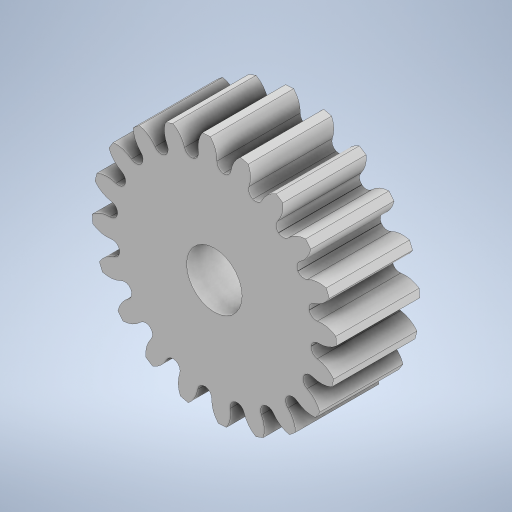
# Autodesk Inventor part: Spur_Gear_20
Saved by Autodesk Inventor 2024 (Build 280153000, 153)
## iProperties
Created: 2024-10-23
Part Number: Spur_Gear_20
Material: Generic
Document SubType Name: Modeling
Designer: Yash Purswani
Density: 1 g/cm^3
Appearance: Default
Author: Yash Purswani
Autodesk Inventor part; units mm, degrees
ref_plane "YZ Plane" through (0, 0, 0) normal (1, 0, 0) x (0, 1, 0)
ref_plane "XZ Plane" through (0, 0, 0) normal (0, 1, 0) x (-1, 0, 0)
ref_plane "XY Plane" through (0, 0, 0) normal (0, 0, 1) x (1, 0, 0)
sketch "Sketch1" plane through (0, 0, 0) normal (0, 0, 1) x (1, 0, 0)
  line L0 (-0.0011, 22.0023) -> (-0.0011, 20.9337)
  arc A0 (0.4688, 18.788) -> (-0.7145, 21.9884) centre (-4.1398, 18.903) ccw
  arc A1 (-2.1725, 21.8925) -> (-2.8834, 18.5713) centre (1.6629, 19.3348) ccw
  arc A2 (-3.8684, 17.0671) -> (-2.8834, 18.5713) centre (-4.1544, 18.3289) ccw
  arc A3 (0.4688, 18.788) -> (1.6392, 17.4231) centre (1.7604, 18.7112) ccw
  arc A4 (-8.8313, 20.1496) -> (-8.4812, 16.7714) centre (-4.3933, 18.9023) ccw
  arc A5 (-5.36, 18.0133) -> (-7.4743, 20.6914) centre (-9.7785, 16.6986) ccw
  arc A6 (-5.36, 18.0133) -> (-3.8251, 17.0768) centre (-4.1079, 18.3394) ccw
  arc A7 (-8.9531, 15.0364) -> (-8.4812, 16.7714) centre (-9.615, 16.1481) ccw
  arc A8 (-14.6257, 16.4344) -> (-13.2487, 13.3297) centre (-10.0194, 16.6196) ccw
  arc A9 (-10.6641, 15.4754) -> (-13.5025, 17.369) centre (-14.4601, 12.8596) ccw
  arc A10 (-10.6641, 15.4754) -> (-8.9149, 15.059) centre (-9.574, 16.1724) ccw
  arc A11 (-13.1614, 11.5338) -> (-13.2487, 13.3297) centre (-14.1344, 12.3865) ccw
  arc A12 (-18.9883, 11.1105) -> (-16.7194, 8.5832) centre (-14.6647, 12.71) ccw
  arc A13 (-14.9243, 11.4226) -> (-18.209, 12.3464) centre (-17.7262, 7.7618) ccw
  arc A14 (-14.9243, 11.4226) -> (-13.1321, 11.5671) centre (-14.103, 12.4223) ccw
  arc A15 (-16.0813, 6.9022) -> (-16.7194, 8.5832) centre (-17.2703, 7.4125) ccw
  arc A16 (-21.4923, 4.699) -> (-18.5534, 2.9965) centre (-17.8746, 7.5563) ccw
  arc A17 (-17.7236, 6.2517) -> (-21.133, 6.1153) centre (-19.2571, 1.9042) ccw
  arc A18 (-17.7236, 6.2517) -> (-16.0638, 6.943) centre (-17.2515, 7.4563) ccw
  arc A19 (-17.4272, 1.595) -> (-18.5534, 2.9965) centre (-18.7156, 1.7129) ccw
  arc A20 (-21.8925, -2.1725) -> (-18.5713, -2.8834) centre (-19.3348, 1.6629) ccw
  arc A21 (-18.788, 0.4688) -> (-21.9884, -0.7145) centre (-18.903, -4.1398) ccw
  arc A22 (-18.788, 0.4688) -> (-17.4231, 1.6392) centre (-18.7112, 1.7604) ccw
  arc A23 (-17.0671, -3.8684) -> (-18.5713, -2.8834) centre (-18.3289, -4.1544) ccw
  arc A24 (-20.1496, -8.8313) -> (-16.7714, -8.4812) centre (-18.9023, -4.3933) ccw
  arc A25 (-18.0133, -5.36) -> (-20.6914, -7.4743) centre (-16.6986, -9.7785) ccw
  arc A26 (-18.0133, -5.36) -> (-17.0768, -3.8251) centre (-18.3394, -4.1079) ccw
  arc A27 (-15.0364, -8.9531) -> (-16.7714, -8.4812) centre (-16.1481, -9.615) ccw
  arc A28 (-16.4344, -14.6257) -> (-13.3297, -13.2487) centre (-16.6196, -10.0194) ccw
  arc A29 (-15.4754, -10.6641) -> (-17.369, -13.5025) centre (-12.8596, -14.4601) ccw
  arc A30 (-15.4754, -10.6641) -> (-15.059, -8.9149) centre (-16.1724, -9.574) ccw
  arc A31 (-11.5338, -13.1614) -> (-13.3297, -13.2487) centre (-12.3865, -14.1344) ccw
  arc A32 (-11.1105, -18.9883) -> (-8.5832, -16.7194) centre (-12.71, -14.6647) ccw
  arc A33 (-11.4226, -14.9243) -> (-12.3464, -18.209) centre (-7.7618, -17.7262) ccw
  arc A34 (-11.4226, -14.9243) -> (-11.5671, -13.1321) centre (-12.4223, -14.103) ccw
  arc A35 (-6.9022, -16.0813) -> (-8.5832, -16.7194) centre (-7.4125, -17.2703) ccw
  arc A36 (-4.699, -21.4923) -> (-2.9965, -18.5534) centre (-7.5563, -17.8746) ccw
  arc A37 (-6.2517, -17.7236) -> (-6.1153, -21.133) centre (-1.9042, -19.2571) ccw
  arc A38 (-6.2517, -17.7236) -> (-6.943, -16.0638) centre (-7.4563, -17.2515) ccw
  arc A39 (-1.595, -17.4272) -> (-2.9965, -18.5534) centre (-1.7129, -18.7156) ccw
  arc A40 (2.1725, -21.8925) -> (2.8834, -18.5713) centre (-1.6629, -19.3348) ccw
  arc A41 (-0.4688, -18.788) -> (0.7145, -21.9884) centre (4.1398, -18.903) ccw
  arc A42 (-0.4688, -18.788) -> (-1.6392, -17.4231) centre (-1.7604, -18.7112) ccw
  arc A43 (3.8684, -17.0671) -> (2.8834, -18.5713) centre (4.1544, -18.3289) ccw
  arc A44 (8.8313, -20.1496) -> (8.4812, -16.7714) centre (4.3933, -18.9023) ccw
  arc A45 (5.36, -18.0133) -> (7.4743, -20.6914) centre (9.7785, -16.6986) ccw
  arc A46 (5.36, -18.0133) -> (3.8251, -17.0768) centre (4.1079, -18.3394) ccw
  arc A47 (8.9531, -15.0364) -> (8.4812, -16.7714) centre (9.615, -16.1481) ccw
  arc A48 (14.6257, -16.4344) -> (13.2487, -13.3297) centre (10.0194, -16.6196) ccw
  arc A49 (10.6641, -15.4754) -> (13.5025, -17.369) centre (14.4601, -12.8596) ccw
  arc A50 (10.6641, -15.4754) -> (8.9149, -15.059) centre (9.574, -16.1724) ccw
  arc A51 (13.1614, -11.5338) -> (13.2487, -13.3297) centre (14.1344, -12.3865) ccw
  arc A52 (18.9883, -11.1105) -> (16.7194, -8.5832) centre (14.6647, -12.71) ccw
  arc A53 (14.9243, -11.4226) -> (18.209, -12.3464) centre (17.7262, -7.7618) ccw
  arc A54 (14.9243, -11.4226) -> (13.1321, -11.5671) centre (14.103, -12.4223) ccw
  arc A55 (16.0813, -6.9022) -> (16.7194, -8.5832) centre (17.2703, -7.4125) ccw
  arc A56 (21.4923, -4.699) -> (18.5534, -2.9965) centre (17.8746, -7.5563) ccw
  arc A57 (17.7236, -6.2517) -> (21.133, -6.1153) centre (19.2571, -1.9042) ccw
  arc A58 (17.7236, -6.2517) -> (16.0638, -6.943) centre (17.2515, -7.4563) ccw
  arc A59 (17.4272, -1.595) -> (18.5534, -2.9965) centre (18.7156, -1.7129) ccw
  arc A60 (21.8925, 2.1725) -> (18.5713, 2.8834) centre (19.3348, -1.6629) ccw
  arc A61 (18.788, -0.4688) -> (21.9884, 0.7145) centre (18.903, 4.1398) ccw
  arc A62 (18.788, -0.4688) -> (17.4231, -1.6392) centre (18.7112, -1.7604) ccw
  arc A63 (17.0671, 3.8684) -> (18.5713, 2.8834) centre (18.3289, 4.1544) ccw
  arc A64 (20.1496, 8.8313) -> (16.7714, 8.4812) centre (18.9023, 4.3933) ccw
  arc A65 (18.0133, 5.36) -> (20.6914, 7.4743) centre (16.6986, 9.7785) ccw
  arc A66 (18.0133, 5.36) -> (17.0768, 3.8251) centre (18.3394, 4.1079) ccw
  arc A67 (15.0364, 8.9531) -> (16.7714, 8.4812) centre (16.1481, 9.615) ccw
  arc A68 (16.4344, 14.6257) -> (13.3297, 13.2487) centre (16.6196, 10.0194) ccw
  arc A69 (15.4754, 10.6641) -> (17.369, 13.5025) centre (12.8596, 14.4601) ccw
  arc A70 (15.4754, 10.6641) -> (15.059, 8.9149) centre (16.1724, 9.574) ccw
  arc A71 (11.5338, 13.1614) -> (13.3297, 13.2487) centre (12.3865, 14.1344) ccw
  arc A72 (11.1105, 18.9883) -> (8.5832, 16.7194) centre (12.71, 14.6647) ccw
  arc A73 (11.4226, 14.9243) -> (12.3464, 18.209) centre (7.7618, 17.7262) ccw
  arc A74 (11.4226, 14.9243) -> (11.5671, 13.1321) centre (12.4223, 14.103) ccw
  arc A75 (6.9022, 16.0813) -> (8.5832, 16.7194) centre (7.4125, 17.2703) ccw
  arc A76 (4.699, 21.4923) -> (2.9965, 18.5534) centre (7.5563, 17.8746) ccw
  arc A77 (6.2517, 17.7236) -> (6.1153, 21.133) centre (1.9042, 19.2571) ccw
  arc A78 (6.2517, 17.7236) -> (6.943, 16.0638) centre (7.4563, 17.2515) ccw
  arc A79 (1.595, 17.4272) -> (2.9965, 18.5534) centre (1.7129, 18.7156) ccw
  arc A80 (20.6914, 7.4743) -> (20.1496, 8.8313) centre (0, 0) ccw
  arc A81 (-17.0768, -3.8251) -> (-17.0671, -3.8684) centre (0, 0) ccw
  arc A82 (-17.4231, 1.6392) -> (-17.4272, 1.595) centre (0, 0) ccw
  arc A83 (-16.0638, 6.943) -> (-16.0813, 6.9022) centre (0, 0) ccw
  arc A84 (-13.1321, 11.5671) -> (-13.1614, 11.5338) centre (0, 0) ccw
  arc A85 (17.4231, -1.6392) -> (17.4272, -1.595) centre (0, 0) ccw
  arc A86 (17.0768, 3.8251) -> (17.0671, 3.8684) centre (0, 0) ccw
  arc A87 (15.059, 8.9149) -> (15.0364, 8.9531) centre (0, 0) ccw
  arc A88 (11.5671, 13.1321) -> (11.5338, 13.1614) centre (0, 0) ccw
  arc A89 (-0.0011, 22) -> (-2.1725, 21.8925) centre (0, 0) ccw
  arc A90 (6.1153, 21.133) -> (4.699, 21.4923) centre (0, 0) ccw
  arc A91 (12.3464, 18.209) -> (11.1105, 18.9883) centre (0, 0) ccw
  arc A92 (17.369, 13.5025) -> (16.4344, 14.6257) centre (0, 0) ccw
  arc A93 (20.6914, 7.4743) -> (20.1496, 8.8313) centre (0, 0) ccw
  arc A94 (21.9884, 0.7145) -> (21.8925, 2.1725) centre (0, 0) ccw
  arc A95 (-7.4743, 20.6914) -> (-8.8313, 20.1496) centre (0, 0) ccw
  arc A96 (-13.5025, 17.369) -> (-14.6257, 16.4344) centre (0, 0) ccw
  arc A97 (13.5025, -17.369) -> (14.6257, -16.4344) centre (0, 0) ccw
  arc A98 (7.4743, -20.6914) -> (8.8313, -20.1496) centre (0, 0) ccw
  arc A99 (0.7145, -21.9884) -> (2.1725, -21.8925) centre (0, 0) ccw
  arc A100 (18.209, -12.3464) -> (18.9883, -11.1105) centre (0, 0) ccw
  arc A101 (21.133, -6.1153) -> (21.4923, -4.699) centre (0, 0) ccw
  arc A102 (-18.209, 12.3464) -> (-18.9883, 11.1105) centre (0, 0) ccw
  arc A103 (-6.1153, -21.133) -> (-4.699, -21.4923) centre (0, 0) ccw
  arc A104 (-21.133, 6.1153) -> (-21.4923, 4.699) centre (0, 0) ccw
  arc A105 (-21.9884, -0.7145) -> (-21.8925, -2.1725) centre (0, 0) ccw
  arc A106 (-20.6914, -7.4743) -> (-20.1496, -8.8313) centre (0, 0) ccw
  arc A107 (-17.369, -13.5025) -> (-16.4344, -14.6257) centre (0, 0) ccw
  arc A108 (-12.3464, -18.209) -> (-11.1105, -18.9883) centre (0, 0) ccw
  circle A109 centre (0, 0) radius 5
  point P0 (-3.8468, 17.0722)
  point P1 (-8.9341, 15.0479)
  point P2 (-13.1469, 11.5506)
  point P3 (-16.0728, 6.9227)
  point P4 (-21.133, 6.1153)
  point P5 (-17.4253, 1.6171)
  point P6 (-21.9884, -0.7145)
  point P7 (-17.0722, -3.8468)
  point P8 (-15.0479, -8.9341)
  point P9 (-17.369, -13.5025)
  point P10 (-11.5506, -13.1469)
  point P11 (-6.9227, -16.0728)
  point P12 (-1.6171, -17.4253)
  point P13 (3.8468, -17.0722)
  point P14 (8.9341, -15.0479)
  point P15 (13.1469, -11.5506)
  point P16 (18.209, -12.3464)
  point P17 (16.0728, -6.9227)
  point P18 (17.4253, -1.6171)
  point P19 (17.0722, 3.8468)
  point P20 (15.0479, 8.9341)
  point P21 (11.5506, 13.1469)
  point P22 (6.9227, 16.0728)
  point P23 (1.6171, 17.4253)
  point P24 (-0.7145, 21.9884)
  dimension "d4" = 1.0686
  dimension "d10" = 360
  dimension "d12" = 10
  constraints: 218 point on circle, 110 centre point, 3 coincident, 2 end point, 1 point on line, 1 vertical, 281 other
  measures "d4" distance of L0.start L0.end
  measures "d12" diameter of A109
extrude "Extrusion1" add sketch "Sketch1" along normal blind 15 contours A0 A3 A79 A76 A90 A77 A78 A75 A72 A91 A73 A74 A71 A68 A92 A69 A70 A67 A64 A80 A65 A66 A63 A60 A94 A61 A62 A59 A56 A101 A57 A58 A55 A52 A100 A53 A54 A51 A48 A97 A49 A50 A47 A44 A98 A45 A46 A43 A40 A99 A41 A42 A39 A36 A103 A37 A38 A35 A32 A108 A33 A34 A31 A28 A107 A29 A30 A27 A24 A106 A25 A26 A23 A20 A105 A21 A22 A19 A16 A104 A17 A18 A15 A12 A102 A13 A14 A11 A8 A96 A9 A10 A7 A4 A95 A5 A6 A2 A1 A89
body "Solid1"
